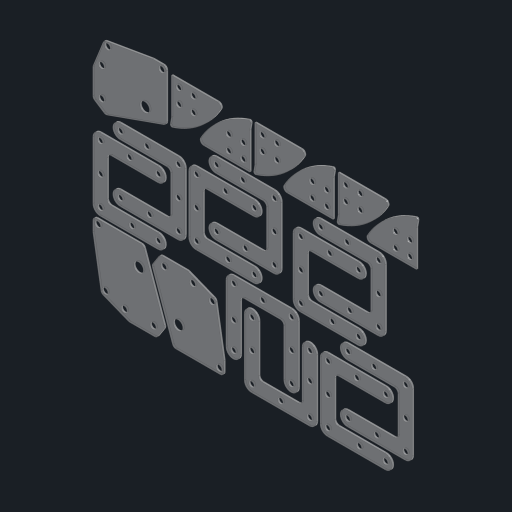
# Autodesk Inventor part: plastic
Saved by Autodesk Inventor 2023 (Build 270158000, 158)
## iProperties
Created: 2023-05-13
Part Number: plastic
Material: Polycarbonate, Clear
Document SubType Name: Modeling
Designer: reima
Density: 1.2 g/cm^3
Appearance: Polycarbonate - Clear
Author: reima
Autodesk Inventor part; units mm, degrees
ref_plane "YZ Plane" through (0, 0, 0) normal (1, 0, 0) x (0, 1, 0)
ref_plane "XZ Plane" through (0, 0, 0) normal (0, 1, 0) x (-1, 0, 0)
ref_plane "XY Plane" through (0, 0, 0) normal (0, 0, 1) x (1, 0, 0)
sketch "newpolytrackers sketch" plane through (0, 0, 0) normal (0, 0, 1) x (1, 0, 0)
  circle A0 centre (46.6055, 51.9778) radius 4.191
  circle A1 centre (10.668, 66.7098) radius 2.54
  circle A2 centre (59.2992, 13.8799) radius 2.54
  circle A3 centre (33.8992, 13.8672) radius 2.54
  circle A4 centre (17.0314, 19.2442) radius 2.54
  arc A5 (13.4092, 17.8242) -> (15.3646, 15.4108) centre (16.5386, 18.3608) ccw
  line L0 (13.4092, 17.8242) -> (6.35, 58.9949)
  line L1 (6.35, 58.9949) -> (6.35, 67.8528)
  arc A6 (9.525, 71.0278) -> (6.35, 67.8528) centre (9.525, 67.8528) ccw
  line L2 (9.525, 71.0278) -> (48.5612, 71.0278)
  arc A7 (51.5544, 68.9118) -> (48.5612, 71.0278) centre (48.5612, 67.8528) ccw
  line L3 (51.5544, 68.9118) -> (69.2142, 18.996)
  arc A8 (68.8848, 16.2093) -> (69.2142, 18.996) centre (66.221, 17.937) ccw
  line L4 (68.8848, 16.2093) -> (63.4289, 7.7973)
  arc A9 (60.7652, 6.35) -> (63.4289, 7.7973) centre (60.7652, 9.525) ccw
  line L5 (60.7652, 6.35) -> (38.7423, 6.35)
  arc A10 (37.5684, 6.575) -> (38.7423, 6.35) centre (38.7423, 9.525) ccw
  line L6 (37.5684, 6.575) -> (15.3646, 15.4108)
  constraints: 14 end point, 12 point on circle, 11 centre point
extrude "newpolytrackers extrude" add sketch "newpolytrackers sketch" along normal blind 1.5875
sketch "frontgusset sketch" plane through (0, 0, 0) normal (0, 0, 1) x (1, 0, 0)
  circle A0 centre (38.1, 131.3529) radius 2.3368
  circle A1 centre (40.4368, 80.5529) radius 2.3368
  circle A2 centre (12.7, 105.9529) radius 2.3368
  circle A3 centre (12.7, 131.3528) radius 2.3114
  circle A4 centre (63.5, 131.3529) radius 2.3114
  circle A5 centre (12.7, 80.5529) radius 2.3114
  circle A6 centre (63.5, 80.5529) radius 2.3114
  arc A7 (6.35, 80.5529) -> (12.7, 74.2029) centre (12.7, 80.5529) ccw
  line L0 (6.35, 80.5529) -> (6.35, 131.3528)
  arc A8 (12.7, 137.7029) -> (6.35, 131.3528) centre (12.7, 131.3528) ccw
  line L1 (12.7, 137.7029) -> (63.5, 137.7029)
  arc A9 (63.5, 125.0029) -> (63.5, 137.7029) centre (63.5, 131.3529) ccw
  line L2 (63.5, 125.0029) -> (22.225, 125.0028)
  arc A10 (22.225, 125.0028) -> (19.05, 121.8279) centre (22.225, 121.8278) ccw
  line L3 (19.05, 121.8279) -> (19.05, 90.0779)
  arc A11 (19.05, 90.0779) -> (22.225, 86.9029) centre (22.225, 90.0779) ccw
  line L4 (22.225, 86.9029) -> (63.5, 86.9029)
  arc A12 (63.5, 74.2029) -> (63.5, 86.9029) centre (63.5, 80.5529) ccw
  line L5 (63.5, 74.2029) -> (12.7, 74.2029)
  constraints: 13 centre point, 12 end point, 12 point on circle
extrude "frontgusset extrude" add sketch "frontgusset sketch" along normal blind 1.5875 separate body
sketch "frontgusset (#2) sketch" plane through (0, 0, 0) normal (0, 0, 1) x (1, 0, 0)
  circle A0 centre (55.6693, 96.6411) radius 2.3368
  circle A1 centre (53.3325, 147.4411) radius 2.3368
  circle A2 centre (81.0693, 122.0411) radius 2.3368
  circle A3 centre (81.0693, 96.6411) radius 2.3114
  circle A4 centre (30.2693, 96.6411) radius 2.3114
  circle A5 centre (81.0693, 147.4411) radius 2.3114
  circle A6 centre (30.2693, 147.4411) radius 2.3114
  arc A7 (87.4193, 147.4411) -> (81.0693, 153.7911) centre (81.0693, 147.4411) ccw
  line L0 (87.4193, 147.4411) -> (87.4193, 96.6411)
  arc A8 (81.0693, 90.2911) -> (87.4193, 96.6411) centre (81.0693, 96.6411) ccw
  line L1 (81.0693, 90.2911) -> (30.2693, 90.2911)
  arc A9 (30.2693, 102.9911) -> (30.2693, 90.2911) centre (30.2693, 96.6411) ccw
  line L2 (30.2693, 102.9911) -> (71.5443, 102.9911)
  arc A10 (71.5443, 102.9911) -> (74.7193, 106.1661) centre (71.5443, 106.1661) ccw
  line L3 (74.7193, 106.1661) -> (74.7193, 137.9161)
  arc A11 (74.7193, 137.9161) -> (71.5443, 141.0911) centre (71.5443, 137.9161) ccw
  line L4 (71.5443, 141.0911) -> (30.2693, 141.0911)
  arc A12 (30.2693, 153.7911) -> (30.2693, 141.0911) centre (30.2693, 147.4411) ccw
  line L5 (30.2693, 153.7911) -> (81.0693, 153.7911)
  constraints: 13 centre point, 12 end point, 12 point on circle
extrude "frontgusset (#2) extrude" add sketch "frontgusset (#2) sketch" along normal blind 1.5875 separate body
sketch "newpolytrackers (#2) sketch" plane through (0, 0, 0) normal (0, 0, 1) x (1, 0, 0)
  circle A0 centre (51.9778, 176.7098) radius 4.191
  circle A1 centre (66.7098, 212.6473) radius 2.54
  circle A2 centre (13.8799, 164.0161) radius 2.54
  circle A3 centre (13.8672, 189.4161) radius 2.54
  circle A4 centre (19.2442, 206.2839) radius 2.54
  arc A5 (17.8242, 209.9061) -> (15.4108, 207.9507) centre (18.3608, 206.7767) ccw
  line L0 (17.8242, 209.9061) -> (58.9949, 216.9653)
  line L1 (58.9949, 216.9653) -> (67.8528, 216.9653)
  arc A6 (71.0278, 213.7903) -> (67.8528, 216.9653) centre (67.8528, 213.7903) ccw
  line L2 (71.0278, 213.7903) -> (71.0278, 174.7541)
  arc A7 (68.9118, 171.7609) -> (71.0278, 174.7541) centre (67.8528, 174.7541) ccw
  line L3 (68.9118, 171.7609) -> (18.9959, 154.1011)
  arc A8 (16.2093, 154.4305) -> (18.9959, 154.1011) centre (17.937, 157.0943) ccw
  line L4 (16.2093, 154.4305) -> (7.7973, 159.8864)
  arc A9 (6.35, 162.5501) -> (7.7973, 159.8864) centre (9.525, 162.5501) ccw
  line L5 (6.35, 162.5501) -> (6.35, 184.573)
  arc A10 (6.575, 185.7469) -> (6.35, 184.573) centre (9.525, 184.573) ccw
  line L6 (6.575, 185.7469) -> (15.4108, 207.9507)
  constraints: 14 end point, 12 point on circle, 11 centre point
extrude "newpolytrackers (#2) extrude" add sketch "newpolytrackers (#2) sketch" along normal blind 1.5875 separate body
sketch "newpolytrackers (#3) sketch" plane through (0, 0, 0) normal (0, 0, 1) x (1, 0, 0)
  circle A0 centre (81.2563, 25.4) radius 4.191
  circle A1 centre (117.1939, 10.668) radius 2.54
  circle A2 centre (68.5626, 63.4979) radius 2.54
  circle A3 centre (93.9626, 63.5106) radius 2.54
  circle A4 centre (110.8305, 58.1337) radius 2.54
  arc A5 (114.4526, 59.5536) -> (112.4972, 61.9671) centre (111.3233, 59.0171) ccw
  line L0 (114.4526, 59.5536) -> (121.5118, 18.3829)
  line L1 (121.5118, 18.3829) -> (121.5119, 9.525)
  arc A6 (118.3369, 6.35) -> (121.5119, 9.525) centre (118.3369, 9.525) ccw
  line L2 (118.3369, 6.35) -> (79.3006, 6.35)
  arc A7 (76.3074, 8.466) -> (79.3006, 6.35) centre (79.3006, 9.525) ccw
  line L3 (76.3074, 8.466) -> (58.6477, 58.3819)
  arc A8 (58.9771, 61.1685) -> (58.6477, 58.3819) centre (61.6409, 59.4409) ccw
  line L4 (58.9771, 61.1685) -> (64.4329, 69.5805)
  arc A9 (67.0967, 71.0278) -> (64.4329, 69.5805) centre (67.0967, 67.8528) ccw
  line L5 (67.0967, 71.0278) -> (89.1196, 71.0278)
  arc A10 (90.2935, 70.8028) -> (89.1196, 71.0278) centre (89.1195, 67.8528) ccw
  line L6 (90.2935, 70.8028) -> (112.4972, 61.9671)
  constraints: 14 end point, 12 point on circle, 11 centre point
extrude "newpolytrackers (#3) extrude" add sketch "newpolytrackers (#3) sketch" along normal blind 1.5875 separate body
sketch "frontgusset (#3) sketch" plane through (0, 0, 0) normal (0, 0, 1) x (1, 0, 0)
  circle A0 centre (122.3443, 147.7443) radius 2.3368
  circle A1 centre (124.6811, 96.9443) radius 2.3368
  circle A2 centre (96.9443, 122.3443) radius 2.3368
  circle A3 centre (96.9443, 147.7443) radius 2.3114
  circle A4 centre (147.7443, 147.7443) radius 2.3114
  circle A5 centre (96.9443, 96.9443) radius 2.3114
  circle A6 centre (147.7443, 96.9443) radius 2.3114
  arc A7 (90.5943, 96.9443) -> (96.9443, 90.5943) centre (96.9443, 96.9443) ccw
  line L0 (90.5943, 96.9443) -> (90.5943, 147.7443)
  arc A8 (96.9443, 154.0943) -> (90.5943, 147.7443) centre (96.9443, 147.7443) ccw
  line L1 (96.9443, 154.0943) -> (147.7443, 154.0943)
  arc A9 (147.7443, 141.3943) -> (147.7443, 154.0943) centre (147.7443, 147.7443) ccw
  line L2 (147.7443, 141.3943) -> (106.4693, 141.3943)
  arc A10 (106.4693, 141.3943) -> (103.2943, 138.2193) centre (106.4693, 138.2193) ccw
  line L3 (103.2943, 138.2193) -> (103.2943, 106.4693)
  arc A11 (103.2943, 106.4693) -> (106.4693, 103.2943) centre (106.4693, 106.4693) ccw
  line L4 (106.4693, 103.2943) -> (147.7443, 103.2943)
  arc A12 (147.7443, 90.5943) -> (147.7443, 103.2943) centre (147.7443, 96.9443) ccw
  line L5 (147.7443, 90.5943) -> (96.9443, 90.5943)
  constraints: 13 centre point, 12 end point, 12 point on circle
extrude "frontgusset (#3) extrude" add sketch "frontgusset (#3) sketch" along normal blind 1.5875 separate body
sketch "sleds sketch" plane through (0, 0, 0) normal (0, 0, 1) x (1, 0, 0)
  circle A0 centre (81.6254, 206.159) radius 2.3114
  circle A1 centre (81.6254, 193.459) radius 2.3114
  circle A2 centre (94.3254, 193.459) radius 2.3114
  circle A3 centre (94.3254, 206.159) radius 2.3114
  line L0 (75.3849, 212.7603) -> (115.9063, 212.7603)
  arc A4 (118.862, 208.4257) -> (115.9063, 212.7603) centre (115.9063, 209.5853) ccw
  arc A5 (76.459, 173.4361) -> (118.862, 208.4257) centre (53.0641, 244.9761) ccw
  arc A6 (74.4022, 175.2207) -> (76.459, 173.4361) centre (75.9656, 174.945) ccw
  line L1 (74.4022, 175.2207) -> (75.3849, 180.7938)
  line L2 (75.3849, 180.7938) -> (75.3849, 212.7603)
  constraints: 7 centre point, 6 end point, 6 point on circle
extrude "sleds extrude" add sketch "sleds sketch" along normal blind 1.5875 separate body
sketch "frontgusset (#4) sketch" plane through (0, 0, 0) normal (0, 0, 1) x (1, 0, 0)
  circle A0 centre (145.7635, 38.1) radius 2.3368
  circle A1 centre (196.5635, 40.4368) radius 2.3368
  circle A2 centre (171.1635, 12.7) radius 2.3368
  circle A3 centre (145.7635, 12.7) radius 2.3114
  circle A4 centre (145.7635, 63.5) radius 2.3114
  circle A5 centre (196.5635, 12.7) radius 2.3114
  circle A6 centre (196.5635, 63.5) radius 2.3114
  arc A7 (196.5635, 6.35) -> (202.9135, 12.7) centre (196.5635, 12.7) ccw
  line L0 (196.5635, 6.35) -> (145.7635, 6.35)
  arc A8 (139.4135, 12.7) -> (145.7635, 6.35) centre (145.7635, 12.7) ccw
  line L1 (139.4135, 12.7) -> (139.4135, 63.5)
  arc A9 (152.1135, 63.5) -> (139.4135, 63.5) centre (145.7635, 63.5) ccw
  line L2 (152.1135, 63.5) -> (152.1135, 22.225)
  arc A10 (152.1135, 22.225) -> (155.2885, 19.05) centre (155.2885, 22.225) ccw
  line L3 (155.2885, 19.05) -> (187.0385, 19.05)
  arc A11 (187.0385, 19.05) -> (190.2135, 22.225) centre (187.0385, 22.225) ccw
  line L4 (190.2135, 22.225) -> (190.2135, 63.5)
  arc A12 (202.9135, 63.5) -> (190.2135, 63.5) centre (196.5635, 63.5) ccw
  line L5 (202.9135, 63.5) -> (202.9135, 12.7)
  constraints: 13 centre point, 12 end point, 12 point on circle
extrude "frontgusset (#4) extrude" add sketch "frontgusset (#4) sketch" along normal blind 1.5875 separate body
sketch "frontgusset (#5) sketch" plane through (0, 0, 0) normal (0, 0, 1) x (1, 0, 0)
  circle A0 centre (180.4753, 55.6693) radius 2.3368
  circle A1 centre (129.6753, 53.3325) radius 2.3368
  circle A2 centre (155.0753, 81.0693) radius 2.3368
  circle A3 centre (180.4753, 81.0693) radius 2.3114
  circle A4 centre (180.4753, 30.2693) radius 2.3114
  circle A5 centre (129.6753, 81.0693) radius 2.3114
  circle A6 centre (129.6753, 30.2693) radius 2.3114
  arc A7 (129.6753, 87.4193) -> (123.3253, 81.0693) centre (129.6753, 81.0693) ccw
  line L0 (129.6753, 87.4193) -> (180.4753, 87.4193)
  arc A8 (186.8253, 81.0693) -> (180.4753, 87.4193) centre (180.4753, 81.0693) ccw
  line L1 (186.8253, 81.0693) -> (186.8253, 30.2693)
  arc A9 (174.1253, 30.2693) -> (186.8253, 30.2693) centre (180.4753, 30.2693) ccw
  line L2 (174.1253, 30.2693) -> (174.1253, 71.5443)
  arc A10 (174.1253, 71.5443) -> (170.9503, 74.7193) centre (170.9503, 71.5443) ccw
  line L3 (170.9503, 74.7193) -> (139.2003, 74.7193)
  arc A11 (139.2003, 74.7193) -> (136.0253, 71.5443) centre (139.2003, 71.5443) ccw
  line L4 (136.0253, 71.5443) -> (136.0253, 30.2693)
  arc A12 (123.3253, 30.2693) -> (136.0253, 30.2693) centre (129.6753, 30.2693) ccw
  line L5 (123.3253, 30.2693) -> (123.3253, 81.0693)
  constraints: 13 centre point, 12 end point, 12 point on circle
extrude "frontgusset (#5) extrude" add sketch "frontgusset (#5) sketch" along normal blind 1.5875 separate body
sketch "frontgusset (#6) sketch" plane through (0, 0, 0) normal (0, 0, 1) x (1, 0, 0)
  circle A0 centre (139.9135, 113.0325) radius 2.3368
  circle A1 centre (137.5767, 163.8325) radius 2.3368
  circle A2 centre (165.3135, 138.4325) radius 2.3368
  circle A3 centre (165.3135, 113.0325) radius 2.3114
  circle A4 centre (114.5135, 113.0325) radius 2.3114
  circle A5 centre (165.3135, 163.8325) radius 2.3114
  circle A6 centre (114.5135, 163.8325) radius 2.3114
  arc A7 (171.6635, 163.8325) -> (165.3135, 170.1825) centre (165.3135, 163.8325) ccw
  line L0 (171.6635, 163.8325) -> (171.6635, 113.0325)
  arc A8 (165.3135, 106.6825) -> (171.6635, 113.0325) centre (165.3135, 113.0325) ccw
  line L1 (165.3135, 106.6825) -> (114.5135, 106.6825)
  arc A9 (114.5135, 119.3825) -> (114.5135, 106.6825) centre (114.5135, 113.0325) ccw
  line L2 (114.5135, 119.3825) -> (155.7885, 119.3825)
  arc A10 (155.7885, 119.3825) -> (158.9635, 122.5575) centre (155.7885, 122.5575) ccw
  line L3 (158.9635, 122.5575) -> (158.9635, 154.3075)
  arc A11 (158.9635, 154.3075) -> (155.7885, 157.4825) centre (155.7885, 154.3075) ccw
  line L4 (155.7885, 157.4825) -> (114.5135, 157.4825)
  arc A12 (114.5135, 170.1825) -> (114.5135, 157.4825) centre (114.5135, 163.8325) ccw
  line L5 (114.5135, 170.1825) -> (165.3135, 170.1825)
  constraints: 13 centre point, 12 end point, 12 point on circle
extrude "frontgusset (#6) extrude" add sketch "frontgusset (#6) sketch" along normal blind 1.5875 separate body
sketch "sleds (#2) sketch" plane through (0, 0, 0) normal (0, 0, 1) x (1, 0, 0)
  circle A0 centre (138.0685, 179.9588) radius 2.3114
  circle A1 centre (138.0685, 192.6588) radius 2.3114
  circle A2 centre (125.3685, 192.6588) radius 2.3114
  circle A3 centre (125.3685, 179.9588) radius 2.3114
  line L0 (144.309, 173.3575) -> (103.7875, 173.3575)
  arc A4 (100.8319, 177.6921) -> (103.7875, 173.3575) centre (103.7875, 176.5325) ccw
  arc A5 (143.2349, 212.6817) -> (100.8319, 177.6921) centre (166.6298, 141.1417) ccw
  arc A6 (145.2917, 210.8972) -> (143.2349, 212.6817) centre (143.7283, 211.1728) ccw
  line L1 (145.2917, 210.8972) -> (144.309, 205.324)
  line L2 (144.309, 205.324) -> (144.309, 173.3575)
  constraints: 7 centre point, 6 end point, 6 point on circle
extrude "sleds (#2) extrude" add sketch "sleds (#2) sketch" along normal blind 1.5875 separate body
sketch "sleds (#3) sketch" plane through (0, 0, 0) normal (0, 0, 1) x (1, 0, 0)
  circle A0 centre (154.9115, 206.7615) radius 2.3114
  circle A1 centre (154.9115, 194.0615) radius 2.3114
  circle A2 centre (167.6116, 194.0615) radius 2.3114
  circle A3 centre (167.6116, 206.7615) radius 2.3114
  line L0 (148.6711, 213.3629) -> (189.1925, 213.3629)
  arc A4 (192.1482, 209.0283) -> (189.1925, 213.3629) centre (189.1925, 210.1879) ccw
  arc A5 (149.7452, 174.0387) -> (192.1482, 209.0283) centre (126.3503, 245.5787) ccw
  arc A6 (147.6884, 175.8232) -> (149.7452, 174.0387) centre (149.2517, 175.5475) ccw
  line L1 (147.6884, 175.8232) -> (148.6711, 181.3963)
  line L2 (148.6711, 181.3963) -> (148.6711, 213.3629)
  constraints: 7 centre point, 6 end point, 6 point on circle
extrude "sleds (#3) extrude" add sketch "sleds (#3) sketch" along normal blind 1.5875 separate body
sketch "frontgusset (#7) sketch" plane through (0, 0, 0) normal (0, 0, 1) x (1, 0, 0)
  circle A0 centre (237.8385, 63.5) radius 2.3368
  circle A1 centre (240.1753, 12.7) radius 2.3368
  circle A2 centre (212.4385, 38.1) radius 2.3368
  circle A3 centre (212.4385, 63.5) radius 2.3114
  circle A4 centre (263.2385, 63.5) radius 2.3114
  circle A5 centre (212.4385, 12.7) radius 2.3114
  circle A6 centre (263.2385, 12.7) radius 2.3114
  arc A7 (206.0885, 12.7) -> (212.4385, 6.35) centre (212.4385, 12.7) ccw
  line L0 (206.0885, 12.7) -> (206.0885, 63.5)
  arc A8 (212.4385, 69.85) -> (206.0885, 63.5) centre (212.4385, 63.5) ccw
  line L1 (212.4385, 69.85) -> (263.2385, 69.85)
  arc A9 (263.2385, 57.15) -> (263.2385, 69.85) centre (263.2385, 63.5) ccw
  line L2 (263.2385, 57.15) -> (221.9635, 57.15)
  arc A10 (221.9635, 57.15) -> (218.7885, 53.975) centre (221.9635, 53.975) ccw
  line L3 (218.7885, 53.975) -> (218.7885, 22.225)
  arc A11 (218.7885, 22.225) -> (221.9635, 19.05) centre (221.9635, 22.225) ccw
  line L4 (221.9635, 19.05) -> (263.2385, 19.05)
  arc A12 (263.2385, 6.35) -> (263.2385, 19.05) centre (263.2385, 12.7) ccw
  line L5 (263.2385, 6.35) -> (212.4385, 6.35)
  constraints: 13 centre point, 12 end point, 12 point on circle
extrude "frontgusset (#7) extrude" add sketch "frontgusset (#7) sketch" along normal blind 1.5875 separate body
sketch "frontgusset (#8) sketch" plane through (0, 0, 0) normal (0, 0, 1) x (1, 0, 0)
  circle A0 centre (213.9319, 146.2632) radius 2.3368
  circle A1 centre (216.2688, 95.4632) radius 2.3368
  circle A2 centre (188.532, 120.8632) radius 2.3368
  circle A3 centre (188.532, 146.2632) radius 2.3114
  circle A4 centre (239.3319, 146.2632) radius 2.3114
  circle A5 centre (188.532, 95.4632) radius 2.3114
  circle A6 centre (239.332, 95.4632) radius 2.3114
  arc A7 (182.1819, 95.4632) -> (188.532, 89.1132) centre (188.532, 95.4632) ccw
  line L0 (182.1819, 95.4632) -> (182.1819, 146.2632)
  arc A8 (188.532, 152.6132) -> (182.1819, 146.2632) centre (188.5319, 146.2632) ccw
  line L1 (188.532, 152.6132) -> (239.3319, 152.6133)
  arc A9 (239.332, 139.9132) -> (239.3319, 152.6133) centre (239.3319, 146.2632) ccw
  line L2 (239.332, 139.9132) -> (198.0569, 139.9132)
  arc A10 (198.0569, 139.9132) -> (194.8819, 136.7382) centre (198.0569, 136.7382) ccw
  line L3 (194.8819, 136.7382) -> (194.8819, 104.9882)
  arc A11 (194.8819, 104.9882) -> (198.0569, 101.8132) centre (198.0569, 104.9882) ccw
  line L4 (198.0569, 101.8132) -> (239.332, 101.8132)
  arc A12 (239.332, 89.1132) -> (239.332, 101.8132) centre (239.332, 95.4632) ccw
  line L5 (239.332, 89.1132) -> (188.532, 89.1132)
  constraints: 13 centre point, 12 end point, 12 point on circle
extrude "frontgusset (#8) extrude" add sketch "frontgusset (#8) sketch" along normal blind 1.5875 separate body
sketch "sleds (#4) sketch" plane through (0, 0, 0) normal (0, 0, 1) x (1, 0, 0)
  circle A0 centre (211.3547, 180.5614) radius 2.3114
  circle A1 centre (211.3547, 193.2614) radius 2.3114
  circle A2 centre (198.6546, 193.2614) radius 2.3114
  circle A3 centre (198.6547, 180.5614) radius 2.3114
  line L0 (217.5952, 173.96) -> (177.0737, 173.96)
  arc A4 (174.1181, 178.2946) -> (177.0737, 173.96) centre (177.0737, 177.135) ccw
  arc A5 (216.521, 213.2842) -> (174.1181, 178.2946) centre (239.916, 141.7442) ccw
  arc A6 (218.5779, 211.4997) -> (216.521, 213.2842) centre (217.0145, 211.7754) ccw
  line L1 (218.5779, 211.4997) -> (217.5952, 205.9265)
  line L2 (217.5952, 205.9265) -> (217.5952, 173.96)
  constraints: 7 centre point, 6 end point, 6 point on circle
extrude "sleds (#4) extrude" add sketch "sleds (#4) sketch" along normal blind 1.5875 separate body
sketch "frontgusset (#9) sketch" plane through (0, 0, 0) normal (0, 0, 1) x (1, 0, 0)
  circle A0 centre (255.4078, 28.7882) radius 2.3368
  circle A1 centre (253.071, 79.5882) radius 2.3368
  circle A2 centre (280.8078, 54.1882) radius 2.3368
  circle A3 centre (280.8078, 28.7882) radius 2.3114
  circle A4 centre (230.0078, 28.7882) radius 2.3114
  circle A5 centre (280.8078, 79.5882) radius 2.3114
  circle A6 centre (230.0078, 79.5882) radius 2.3114
  arc A7 (287.1578, 79.5882) -> (280.8078, 85.9382) centre (280.8078, 79.5882) ccw
  line L0 (287.1578, 79.5882) -> (287.1578, 28.7882)
  arc A8 (280.8078, 22.4382) -> (287.1578, 28.7882) centre (280.8078, 28.7882) ccw
  line L1 (280.8078, 22.4382) -> (230.0078, 22.4382)
  arc A9 (230.0078, 35.1382) -> (230.0078, 22.4382) centre (230.0078, 28.7882) ccw
  line L2 (230.0078, 35.1382) -> (271.2828, 35.1382)
  arc A10 (271.2828, 35.1382) -> (274.4578, 38.3132) centre (271.2828, 38.3132) ccw
  line L3 (274.4578, 38.3132) -> (274.4578, 70.0632)
  arc A11 (274.4578, 70.0632) -> (271.2828, 73.2382) centre (271.2828, 70.0632) ccw
  line L4 (271.2828, 73.2382) -> (230.0078, 73.2382)
  arc A12 (230.0078, 85.9382) -> (230.0078, 73.2382) centre (230.0078, 79.5882) ccw
  line L5 (230.0078, 85.9382) -> (280.8078, 85.9382)
  constraints: 13 centre point, 12 end point, 12 point on circle
extrude "frontgusset (#9) extrude" add sketch "frontgusset (#9) sketch" along normal blind 1.5875 separate body
sketch "frontgusset (#10) sketch" plane through (0, 0, 0) normal (0, 0, 1) x (1, 0, 0)
  circle A0 centre (231.5012, 111.5515) radius 2.3368
  circle A1 centre (229.1644, 162.3515) radius 2.3368
  circle A2 centre (256.9012, 136.9515) radius 2.3368
  circle A3 centre (256.9012, 111.5515) radius 2.3114
  circle A4 centre (206.1012, 111.5515) radius 2.3114
  circle A5 centre (256.9012, 162.3515) radius 2.3114
  circle A6 centre (206.1012, 162.3515) radius 2.3114
  arc A7 (263.2512, 162.3515) -> (256.9012, 168.7015) centre (256.9012, 162.3515) ccw
  line L0 (263.2512, 162.3515) -> (263.2512, 111.5515)
  arc A8 (256.9012, 105.2015) -> (263.2512, 111.5515) centre (256.9012, 111.5515) ccw
  line L1 (256.9012, 105.2015) -> (206.1012, 105.2015)
  arc A9 (206.1012, 117.9015) -> (206.1012, 105.2015) centre (206.1012, 111.5515) ccw
  line L2 (206.1012, 117.9015) -> (247.3762, 117.9015)
  arc A10 (247.3762, 117.9015) -> (250.5512, 121.0765) centre (247.3762, 121.0765) ccw
  line L3 (250.5512, 121.0765) -> (250.5512, 152.8265)
  arc A11 (250.5512, 152.8265) -> (247.3762, 156.0015) centre (247.3762, 152.8265) ccw
  line L4 (247.3762, 156.0015) -> (206.1012, 156.0015)
  arc A12 (206.1012, 168.7015) -> (206.1012, 156.0015) centre (206.1012, 162.3515) ccw
  line L5 (206.1012, 168.7015) -> (256.9012, 168.7015)
  constraints: 13 centre point, 12 end point, 12 point on circle
extrude "frontgusset (#10) extrude" add sketch "frontgusset (#10) sketch" along normal blind 1.5875 separate body
sketch "sleds (#5) sketch" plane through (0, 0, 0) normal (0, 0, 1) x (1, 0, 0)
  circle A0 centre (228.1359, 205.2805) radius 2.3114
  circle A1 centre (228.1359, 192.5805) radius 2.3114
  circle A2 centre (240.836, 192.5805) radius 2.3114
  circle A3 centre (240.836, 205.2805) radius 2.3114
  line L0 (221.8954, 211.8818) -> (262.4169, 211.8818)
  arc A4 (265.3726, 207.5472) -> (262.4169, 211.8818) centre (262.4169, 208.7068) ccw
  arc A5 (222.9696, 172.5576) -> (265.3726, 207.5472) centre (199.5746, 244.0977) ccw
  arc A6 (220.9128, 174.3422) -> (222.9696, 172.5576) centre (222.4761, 174.0665) ccw
  line L1 (220.9128, 174.3422) -> (221.8954, 179.9153)
  line L2 (221.8954, 179.9153) -> (221.8954, 211.8818)
  constraints: 7 centre point, 6 end point, 6 point on circle
extrude "sleds (#5) extrude" add sketch "sleds (#5) sketch" along normal blind 1.5875 separate body
sketch "sleds (#6) sketch" plane through (0, 0, 0) normal (0, 0, 1) x (1, 0, 0)
  circle A0 centre (284.579, 179.0803) radius 2.3114
  circle A1 centre (284.579, 191.7803) radius 2.3114
  circle A2 centre (271.8791, 191.7803) radius 2.3114
  circle A3 centre (271.8791, 179.0803) radius 2.3114
  line L0 (290.8195, 172.479) -> (250.2981, 172.479)
  arc A4 (247.3425, 176.8136) -> (250.2981, 172.479) centre (250.2981, 175.654) ccw
  arc A5 (289.7454, 211.8032) -> (247.3425, 176.8136) centre (313.1403, 140.2632) ccw
  arc A6 (291.8022, 210.0187) -> (289.7454, 211.8032) centre (290.2389, 210.2943) ccw
  line L1 (291.8022, 210.0187) -> (290.8195, 204.4455)
  line L2 (290.8195, 204.4455) -> (290.8195, 172.479)
  constraints: 7 centre point, 6 end point, 6 point on circle
extrude "sleds (#6) extrude" add sketch "sleds (#6) sketch" along normal blind 1.5875 separate body
